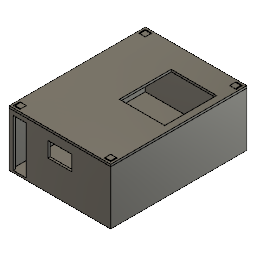
Temperature logger v1 v7 (Autodesk Fusion 360 design; units mm, degrees)
Autodesk Fusion 360 part; units mm, degrees
sketch "Sketch1" plane through (0, 0, 0) normal (0, 1, 0) x (1, 0, 0)
  line L0 (0, 0) -> (45, 0)
  line L1 (45, 0) -> (45, -61)
  line L2 (45, -61) -> (0, -61)
  line L3 (0, -61) -> (0, 0)
  line L4 (-1, 1) -> (46, 1)
  line L5 (46, 1) -> (46, -62)
  line L6 (46, -62) -> (-1, -62)
  line L7 (-1, -62) -> (-1, 1)
  dimension "d1" = 45
  dimension "d2" = 61
  dimension "d3" = 47
  dimension "d4" = 63
  constraint horizontal L0
  constraint vertical L1
  constraint horizontal L2
  constraint vertical L3
  constraint coincident L0.start L3.end
  constraint horizontal L4
  constraint vertical L5
  constraint horizontal L6
  constraint vertical L7
  measures "d1" distance of L0.start L0.end
  measures "d2" distance of L0.start L2.end
  measures "d3" distance of L4.start L4.end
  measures "d4" distance of L4.start L6.end
extrude "Extrude1" add sketch "Sketch1" along normal blind 26 makes body 1
extrude "Extrude2" add sketch "Sketch1" along normal blind 2 contours L0 L1 L2 L3 bodies 1
copy_body "Body->Comp1" bodies 1 removing the originals makes body 2 in component "scatola"
sketch "Sketch2" plane through (0, 0, 62) normal (0, 0, 1) x (1, 0, 0)
  line L0 (-1, 0) -> (46, 0)
  line L1 (46, 0) -> (46, 26)
  line L2 (46, 26) -> (-1, 26)
  line L3 (-1, 26) -> (-1, 0)
  line L4 (1, 24) -> (7, 24)
  line L5 (7, 24) -> (7, 2)
  line L6 (7, 2) -> (1, 2)
  line L7 (1, 2) -> (1, 24)
  line L8 (13, 17) -> (24, 17)
  line L9 (24, 17) -> (24, 10)
  line L10 (24, 10) -> (13, 10)
  line L11 (13, 10) -> (13, 17)
  dimension "d9" = 6
  dimension "d10" = 11
  dimension "d11" = 7
  dimension "d12" = 10
  dimension "d13" = 14
  dimension "d14" = 2
  dimension "d15" = 2
  constraint horizontal L4
  constraint vertical L5
  constraint horizontal L6
  constraint vertical L7
  constraint horizontal L8
  constraint vertical L9
  constraint horizontal L10
  constraint vertical L11
  measures "d9" distance of L4.start L4.end
  measures "d10" distance of L8.start L8.end
  measures "d11" distance of L8.start L10.end
  measures "d12" distance of L0 L10
  measures "d13" distance of L3 L11
  measures "d14" distance of L0 L6
  measures "d15" distance of L3 L7
extrude "Extrude1'" cut sketch "Sketch2" against normal blind 8 contours L4 L5 L6 L7 bodies 2 in component "scatola"
extrude "Extrude2'" cut sketch "Sketch2" against normal blind 4 contours L8 L9 L10 L11 bodies 2 in component "scatola"
extrude "Extrude3" cut 1 faces at (14.6667, 0, 20) along direction (0, 1, 0) blind 1 on bodies 2 bodies 2 in component "scatola"
sketch "Sketch3" plane through (0, 26, 0) normal (0, 1, 0) x (-1, 0, 0)
  line L0 (-45, 61) -> (0, 61)
  line L1 (0, 61) -> (0, 0)
  line L2 (0, 0) -> (-45, 0)
  line L3 (-45, 0) -> (-45, 61)
  line L4 (1, 62) -> (-46, 62)
  line L5 (-46, 62) -> (-46, -1)
  line L6 (-46, -1) -> (1, -1)
  line L7 (1, -1) -> (1, 62)
  line L8 (-46, 62) -> (1, 62)
  line L9 (1, 62) -> (1, -1)
  line L10 (1, -1) -> (-46, -1)
  line L11 (-46, -1) -> (-46, 62)
  line L12 (-46, 62) -> (1, 62)
  line L13 (1, 62) -> (1, -1)
  line L14 (1, -1) -> (-46, -1)
  line L15 (-46, -1) -> (-46, 62)
  line L16 (0, 0) -> (-45, 0)
  line L17 (-45, 0) -> (-45, 25)
  line L18 (-45, 25) -> (0, 25)
  line L19 (0, 25) -> (0, 0)
  line L20 (0, 0) -> (-3, 0)
  line L21 (-3, 0) -> (-3, 3)
  line L22 (-3, 3) -> (0, 3)
  line L23 (0, 3) -> (0, 0)
  line L24 (-45, 0) -> (-42, 0)
  line L25 (-42, 0) -> (-42, 3)
  line L26 (-42, 3) -> (-45, 3)
  line L27 (-45, 3) -> (-45, 0)
  line L28 (-45, 61) -> (-42, 61)
  line L29 (-42, 61) -> (-42, 58)
  line L30 (-42, 58) -> (-45, 58)
  line L31 (-45, 58) -> (-45, 61)
  line L32 (0, 61) -> (-3, 61)
  line L33 (-3, 61) -> (-3, 58)
  line L34 (-3, 58) -> (0, 58)
  line L35 (0, 58) -> (0, 61)
  dimension "d24" = 25
  dimension "d27" = 3
  dimension "d28" = 3
  dimension "d29" = 3
  dimension "d30" = 3
  dimension "d31" = 3
  dimension "d32" = 3
  dimension "d33" = 3
  dimension "d34" = 3
  constraint horizontal L8
  constraint vertical L9
  constraint horizontal L10
  constraint vertical L11
  constraint coincident L6.end L7.start
  constraint coincident L4.end L5.start
  constraint horizontal L12
  constraint vertical L13
  constraint horizontal L14
  constraint vertical L15
  constraint horizontal L16
  constraint vertical L17
  constraint horizontal L18
  constraint vertical L19
  constraint coincident L1.end L2.start
  constraint horizontal L20
  constraint vertical L21
  constraint horizontal L22
  constraint vertical L23
  constraint horizontal L24
  constraint vertical L25
  constraint horizontal L26
  constraint vertical L27
  constraint horizontal L28
  constraint vertical L29
  constraint horizontal L30
  constraint vertical L31
  constraint coincident L0.start L3.end
  constraint horizontal L32
  constraint vertical L33
  constraint horizontal L34
  constraint vertical L35
  constraint coincident L0.end L1.start
  measures "d24" distance of L1.end L18.end
  measures "d27" distance of L1.end L20.end
  measures "d28" distance of L1.end L22.end
  measures "d29" distance of L2.end L24.end
  measures "d30" distance of L2.end L26.end
  measures "d31" distance of L0.start L28.end
  measures "d32" distance of L0.start L30.end
  measures "d33" distance of L0.end L32.end
  measures "d34" distance of L0.end L34.end
extrude "Extrude4" add sketch "Sketch3" along normal blind 3 separate body contours L0 L3 L28 L29 L30 L31 | L0 L1 L32 L33 L34 L35 | L2 L3 L16 L17 L24 L25 L26 L27 | L1 L2 L16 L19 L20 L21 L22 L23 makes body 3 at (0, 27, 2) makes body 4 at (44, 27, 61) makes body 5 at (2, 27, 61) makes body 6 at (43, 27, 3)
extrude "Extrude3'" add sketch "Sketch3" along normal blind 1 separate body contours L0 L3 L28 L29 L30 L31 | L0 L1 L3 L18 L29 L30 L33 L34 | L0 L1 L32 L33 L34 L35 | L4 L5 L6 L7 L8 L9 L10 L11 L12 L13 L14 L15 makes body 7
copy_body "Body->Comp2" bodies 7 removing the originals makes body 8 in component "tappo"
move_body "Move1" bodies 6 5 4 3 to x (1, 0, 0) y (0, 1, 0) z (0, 0, 1) at (0, -2, 0)
combine "Combine1" operation cut target body 8 tool bodies 6 5 4 3 keep tools in component "tappo"
combine "Combine1'" operation add target body 2 tool bodies 3 4 5 6 in component "scatola"
move_face "OffsetFaces1" offset -0.4 8 faces at (0, 26.3333, 60) (0, 26.6667, 1) (1, 26.3333, 0) (1, 26.6667, 61) (44, 26.3333, 61) (45, 26.3333, 59) (45, 26.3333, 1) (43, 26.3333, 0) on bodies 2 in component "scatola"
move_face "MoveFace1" by (4, 5, 0) 4 faces at (20.3333, 10, 61.6667) (13, 12.3333, 61.6667) (16.6667, 17, 61.6667) (24, 14.6667, 61.6667) on bodies 2 in component "scatola"
move_face "OffsetFaces1'" offset 22 1 faces at (0, 26.3333, 16.6667) on bodies 8 in component "tappo"
sketch "Sketch4" plane through (0, 31, 0) normal (0, 1, 0) x (-1, 0, 0)
  line L0 (-45, 58) -> (-45, 61)
  line L1 (-45, 61) -> (-42, 61)
  line L2 (-42, 61) -> (-42, 58)
  line L3 (-42, 58) -> (-45, 58)
  line L4 (0, 58) -> (-3, 58)
  line L5 (-3, 58) -> (-3, 61)
  line L6 (-3, 61) -> (0, 61)
  line L7 (0, 61) -> (0, 58)
  line L8 (-45, 25) -> (-22, 25)
  line L9 (-22, 25) -> (-22, 0)
  line L10 (-22, 0) -> (-45, 0)
  line L11 (-45, 0) -> (-45, 25)
  line L12 (-46, -1) -> (1, -1)
  line L13 (1, -1) -> (1, 62)
  line L14 (1, 62) -> (-46, 62)
  line L15 (-46, 62) -> (-46, -1)
  line L16 (-45, 0) -> (-35, 0)
  line L17 (-35, 0) -> (-35, 10)
  line L18 (-35, 10) -> (-45, 10)
  line L19 (-45, 10) -> (-45, 0)
  dimension "d39" = 10
  dimension "d40" = 10
  constraint horizontal L16
  constraint vertical L17
  constraint horizontal L18
  constraint vertical L19
  constraint coincident L10.end L11.start
  measures "d39" distance of L10.end L16.end
  measures "d40" distance of L10.end L18.end
extrude "Extrude1''" add sketch "Sketch4" against normal blind 1 contours L10 L11 L16 L17 L18 L19 sketch seen with x (1, 0, 0) y (0, 1, 0) z (0, 0, 1) at (0, -4, 0) bodies 8 in component "tappo"
extrude "Extrude2''" add 1 faces at (26.3333, 26.3333, 0) along direction (0, 0, 1) blind 2 on bodies 8 bodies 8 in component "tappo"
extrude "Extrude3''" add 1 faces at (45, 26.6667, 20) along direction (-1, 0, 0) blind 2 on bodies 8 bodies 8 in component "tappo"
combine "Combine2" operation cut target body 8 tool bodies 2 keep tools in component "tappo"
move_face "OffsetFaces2" offset -0.4 2 faces at (1.2667, 26.3333, 0.4) (0.4, 26.3333, 2.1333) on bodies 8 in component "tappo"
move_face "OffsetFaces3" offset -0.4 2 faces at (44.6, 26.3333, 1.2667) (42.8667, 26.3333, 0.4) on bodies 8 in component "tappo"
extrude "Extrude4'" add 1 faces at (26.3333, 26.3333, 2) along direction (0, 0, 1) blind 8 on bodies 8 bodies 8 in component "tappo"
extrude "Extrude5" cut 1 faces at (36, 26.3333, 25) along direction (0, 0, 1) blind 4 on bodies 8 bodies 8 in component "tappo"
extrude "Extrude6" cut 1 faces at (36, 26.3333, 29) along direction (0, 0, 1) blind 5 on bodies 8 bodies 8 in component "tappo"
component "scatola" placed x (1, 0, 0) y (0, 1, 0) z (0, 0, 1) at (0, 0, 0)
component "tappo" placed x (1, 0, 0) y (0, 1, 0) z (0, 0, 1) at (0, 0, 0)
